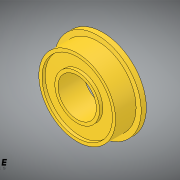
# Autodesk Inventor part: ベアリングフランジ6-12
Saved by Autodesk Inventor 2019 (Build 230136000, 136)
## iProperties
Created: 2019-10-30
Part Number: ベアリングフランジ6-12
Material: 一般
Document SubType Name: Modeling
Designer: tanjihayato
Density: 6.28892 g/cm^3
Appearance: 光沢 - ゴールド
Mass: 1.94 g
Surface Area: 5.2075 cm^2
Volume: 0.308479 cm^3
Author: tanjihayato
Autodesk Inventor part; units mm, degrees
ref_plane "YZ Plane" through (0, 0, 0) normal (1, 0, 0) x (0, 1, 0)
ref_plane "XZ Plane" through (0, 0, 0) normal (0, 1, 0) x (-1, 0, 0)
ref_plane "XY Plane" through (0, 0, 0) normal (0, 0, 1) x (1, 0, 0)
sketch "スケッチ1" plane through (0, 0, 0) normal (0, 0, 1) x (1, 0, 0)
  circle A0 centre (0, 0) radius 6
  circle A1 centre (0, 0) radius 3
  circle A2 centre (0, 0) radius 6.8
  circle A3 centre (0, 0) radius 5.5
  circle A4 centre (0, 0) radius 3.5
  dimension "d0" = 12
  dimension "d1" = 6
  dimension "d4" = 0.8
  dimension "d6" = 0.5
  dimension "d7" = 0.5
  constraints: 5 centre point, 2 coincident
  measures "d0" diameter of A0
  measures "d1" diameter of A1
  measures "d4" radial gap between concentric circles of A0 A2
  measures "d6" radial gap between concentric circles of A0 A3
  measures "d7" radial gap between concentric circles of A1 A4
extrude "押し出し1" add sketch "スケッチ1" along normal blind 0.8 contours A2
extrude "押し出し2" add sketch "スケッチ1" along normal blind 4 contours A0 | A4
extrude "押し出し3" add sketch "スケッチ1" along normal blind 3.5 contours A3
extrude "押し出し5" cut sketch "スケッチ1" along normal blind 0.5 contours A3
